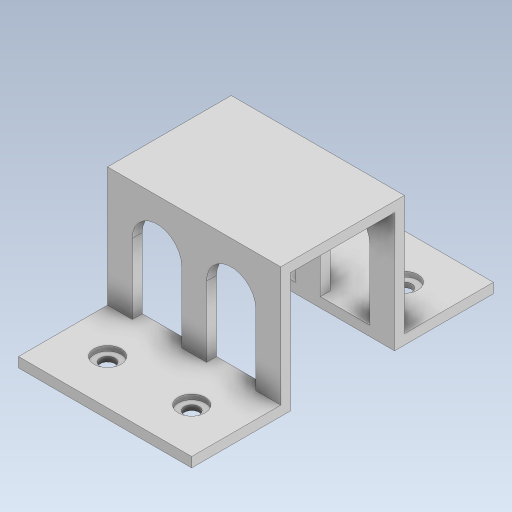
# Autodesk Inventor part: Bracket Motor
Saved by Autodesk Inventor 2023.5 (Build 275446000, 446)
## iProperties
Created: 2025-09-05
Part Number: Bracket Motor
Material: Generic
Document SubType Name: Modeling
Designer: Guntur
Density: 1 g/cm^3
Appearance: Default
Author: Guntur
Autodesk Inventor part; units mm, degrees
ref_plane "YZ Plane" through (0, 0, 0) normal (1, 0, 0) x (0, 1, 0)
ref_plane "XZ Plane" through (0, 0, 0) normal (0, 1, 0) x (-1, 0, 0)
ref_plane "XY Plane" through (0, 0, 0) normal (0, 0, 1) x (1, 0, 0)
sketch "Sketch1" plane through (0, 0, 0) normal (0, 1, 0) x (-1, 0, 0)
  line L0 (0, 0) -> (-35, 0)
  line L1 (-35, 0) -> (-35, -20)
  line L2 (-35, -20) -> (0, -20)
  line L3 (0, -20) -> (0, 0)
  dimension "d0" = 35
  dimension "d1" = 20
  constraints: 8 end point, 2 parallel, 1 horizontal, 1 perpendicular
  measures "d0" distance of L2.end L1.end
  measures "d1" distance of L1.end L0.end
extrude "Extrusion1" add sketch "Sketch1" along normal blind 2
sketch "Sketch2" plane through (0, 2, 0) normal (0, 1, 0) x (1, 0, 0)
  line L0 (0, 20) -> (0, 0) projected
  line L1 (35, 0) -> (35, 20) projected
  line L2 (0, 0) -> (35, 0)
  line L3 (35, 0) -> (35, 2)
  line L4 (35, 2) -> (0, 2)
  line L5 (0, 2) -> (0, 0)
  dimension "d4" = 2
  constraints: 8 end point, 2 parallel, 1 horizontal, 1 perpendicular, 1 point on line
  measures "d4" distance of L3.end L2.end
extrude "Extrusion2" add sketch "Sketch2" along normal blind 24.2
sketch "Sketch3" plane through (0, 0, 0) normal (0, 0, 1) x (1, 0, 0)
  line L0 (0, 0) -> (0, 26.2) projected
  line L1 (35, 0) -> (35, 26.2) projected
  line L2 (0, 26.2) -> (35, 26.2)
  line L3 (35, 26.2) -> (35, 24.2)
  line L4 (35, 24.2) -> (0, 24.2)
  line L5 (0, 24.2) -> (0, 26.2)
  dimension "d7" = 2
  constraints: 8 end point, 2 parallel, 1 horizontal, 1 perpendicular, 1 point on line
  measures "d7" distance of L2.end L3.end
extrude "Extrusion3" add sketch "Sketch3" along normal blind 23
sketch "Sketch4" plane through (0, 24.2, 0) normal (0, -1, 0) x (1, 0, 0)
  line L0 (35, -2) -> (35, 23) projected
  line L1 (0, 0) -> (0, 23) projected
  line L2 (35, 23) -> (0, 23)
  line L3 (0, 23) -> (0, 21)
  line L4 (0, 21) -> (35, 21)
  line L5 (35, 21) -> (35, 23)
  dimension "d10" = 2
  constraints: 8 end point, 2 parallel, 1 horizontal, 1 perpendicular, 1 point on line
  measures "d10" distance of L3.end L2.end
extrude "Extrusion4" add sketch "Sketch4" along normal blind 24.2
sketch "Sketch5" plane through (0, 0, 23) normal (0, 0, 1) x (1, 0, 0)
  line L0 (0, 0) -> (0, 2) projected
  line L1 (35, 2) -> (0, 2) projected
  line L2 (0, 0) -> (35, 0)
  line L3 (35, 0) -> (35, 2)
  line L4 (35, 2) -> (0, 2)
  line L5 (0, 2) -> (0, 0)
  constraints: 8 end point, 2 parallel, 1 horizontal, 1 perpendicular
extrude "Extrusion5" add sketch "Sketch5" along normal blind 18
sketch "Sketch6" plane through (0, 2, 0) normal (0, 1, 0) x (1, 0, 0)
  circle A0 centre (26, 11) radius 1.5
  line L0 (35, 20) -> (0, 20) projected
  line L1 (35, 2) -> (35, 20) projected
  circle A1 centre (9, 11) radius 1.5
  circle A2 centre (26, 11) radius 2.75
  circle A3 centre (9, 11) radius 2.75
  point P0 (0, 0)
  dimension "d15" = 3
  dimension "d16" = 9
  dimension "d17" = 9
  dimension "d18" = 3
  dimension "d19" = 17
  dimension "d20" = 5.5
  dimension "d21" = 5.5
  constraints: 4 centre point, 2 coincident
  measures "d15" diameter of A0
  measures "d16" distance from line of L0 A0.centre
  measures "d17" distance from line of L1 A0.centre
  measures "d18" diameter of A1
  measures "d19" distance of A0.centre A1.centre
  measures "d20" diameter of A2
  measures "d21" diameter of A3
extrude "Extrusion6" cut sketch "Sketch6" against normal blind 2 contours A0 | A1
extrude "Extrusion7" cut sketch "Sketch6" against normal blind 1
sketch "Sketch7" plane through (0, 2, 23) normal (0, 1, 0) x (1, 0, 0)
  circle A0 centre (26, -9) radius 1.5
  line L0 (35, -18) -> (0, -18) projected
  line L1 (35, 0) -> (35, -18) projected
  circle A1 centre (9, -9) radius 1.5
  circle A2 centre (26, -9) radius 2.75
  circle A3 centre (9, -9) radius 2.75
  point P0 (0, 23)
  dimension "d26" = 3
  dimension "d27" = 9
  dimension "d28" = 9
  dimension "d29" = 3
  dimension "d30" = 17
  dimension "d31" = 5.5
  dimension "d32" = 5.5
  constraints: 4 centre point, 2 coincident
  measures "d26" diameter of A0
  measures "d27" distance from line of L0 A0.centre
  measures "d28" distance from line of L1 A0.centre
  measures "d29" diameter of A1
  measures "d30" distance of A1.centre A0.centre
  measures "d31" diameter of A2
  measures "d32" diameter of A3
extrude "Extrusion8" cut sketch "Sketch7" against normal blind 2 contours A0 | A1
extrude "Extrusion9" cut sketch "Sketch7" against normal blind 1
sketch "Sketch8" plane through (35, 2, -2) normal (0, 0, -1) x (-1, 0, 0)
  arc A0 (15, 14.2) -> (5, 14.2) centre (10, 14.2) ccw
  line L0 (0, 24.2) -> (35, 24.2) projected
  line L1 (0, 0) -> (0, 24.2) projected
  line L2 (17.5, 24.2) -> (17.5, 0)
  line L3 (35, 0) -> (0, 0) projected
  line L4 (5, 14.2) -> (5, -0.3272)
  line L5 (15, 14.2) -> (15, 0)
  arc A1 (30, 14.2) -> (20, 14.2) centre (25, 14.2) ccw
  line L6 (30, 14.2) -> (30, -0.3272)
  line L7 (20, 14.2) -> (20, 0)
  point P0 (35, -2)
  point P1 (20, 0)
  point P2 (30, 0)
  point P3 (5, 0)
  dimension "d37" = 10
  dimension "d38" = 10
  dimension "d39" = 10
  constraints: 10 end point, 5 symmetric about line, 4 point on circle, 2 centre point, 2 midpoint, 2 perpendicular, 1 point on line, 1 other
  measures "d37" diameter of A0
  measures "d38" distance from line of L0 A0.centre
  measures "d39" distance from line of L1 A0.centre
extrude "Extrusion10" cut sketch "Sketch8" against normal blind 25 contours L5 L3 L4 A0 | L3 L7 A1 L6
body "Solid1"
